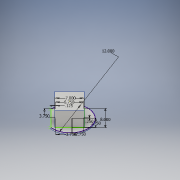
# Autodesk Inventor part: Hermes plate
Saved by Autodesk Inventor 2016 (Build 200138000, 138)
## iProperties
Created: 2016-12-06
Part Number: Hermes plate
Material: Aluminum 6061
Document SubType Name: Modeling
Designer: Ethan
Density: 2.7 g/cm^3
Appearance: Aluminum - Flat
Mass: 3970.64 g
Surface Area: 4553.61 cm^2
Volume: 1470.61 cm^3
Author: Ethan
Autodesk Inventor part; units mm, degrees
ref_plane "YZ Plane" through (0, 0, 0) normal (1, 0, 0) x (0, 1, 0)
ref_plane "XZ Plane" through (0, 0, 0) normal (0, 1, 0) x (-1, 0, 0)
ref_plane "XY Plane" through (0, 0, 0) normal (0, 0, 1) x (1, 0, 0)
sketch "Sketch1" plane through (0, 0, 0) normal (0, 1, 0) x (-1, 0, 0)
  arc A0 (13.4296, 151.8071) -> (151.8071, 13.4296) centre (0, 0) ccw
  line L0 (13.4296, 151.8071) -> (151.8071, 13.4296)
  dimension "d0" = 304.8
  constraints: 2 end point, 2 point on circle, 1 centre point, 1 coincident
  measures "d0" diameter of A0
sketch "Sketch2" plane through (0, 0, 0) normal (0, 1, 0) x (-1, 0, 0)
  line L0 (-4.2626, 135.0266) -> (-129.9862, 9.3031)
  line L1 (-129.9862, 9.3031) -> (13.6979, -134.381)
  line L2 (13.6979, -134.381) -> (139.4215, -8.6575)
  line L3 (139.4215, -8.6575) -> (-4.2626, 135.0266)
  line L4 (-4.2626, 135.0266) -> (-76.1046, 63.1846)
  line L5 (-76.1046, 63.1846) -> (-4.2626, -8.6575)
  line L6 (-4.2626, -8.6575) -> (67.5795, 63.1846)
  line L7 (67.5795, 63.1846) -> (-4.2626, 135.0266)
  line L8 (-129.9862, 9.3031) -> (-76.1046, 63.1846)
  line L9 (-76.1046, 63.1846) -> (-4.2626, -8.6575)
  line L10 (-4.2626, -8.6575) -> (-58.1441, -62.539)
  line L11 (-58.1441, -62.539) -> (-129.9862, 9.3031)
  line L12 (-4.2626, 130.5365) -> (-71.6145, 63.1846)
  line L13 (-71.6145, 63.1846) -> (-4.2626, -4.1673)
  line L14 (-4.2626, -4.1673) -> (63.0893, 63.1846)
  line L15 (63.0893, 63.1846) -> (-4.2626, 130.5365)
  line L16 (-125.496, 9.3031) -> (-76.1046, 58.6945)
  line L17 (-76.1046, 58.6945) -> (-8.7527, -8.6575)
  line L18 (-8.7527, -8.6575) -> (-58.1441, -58.0489)
  line L19 (-58.1441, -58.0489) -> (-125.496, 9.3031)
  line L20 (67.5795, 58.6945) -> (-53.654, -62.539)
  line L21 (-53.654, -62.539) -> (13.6979, -129.8909)
  line L22 (13.6979, -129.8909) -> (134.9314, -8.6575)
  line L23 (134.9314, -8.6575) -> (67.5795, 58.6945)
  point P0 (0, 0)
  point P1 (4.7177, 0.3228)
  dimension "d42" = 203.2
  dimension "d43" = 177.8
  dimension "d44" = 3.175
  dimension "d45" = 6.35
  dimension "d46" = 95.25
  dimension "d47" = 171.45
  dimension "d48" = 95.25
  dimension "d49" = 69.85
  dimension "d50" = 95.25
  constraints: 48 end point, 12 parallel, 6 perpendicular
  measures "d42" distance of L0.end L1.end
  measures "d43" distance of L1.end L2.end
  measures "d44" distance between parallel lines of L3 L23
  measures "d45" distance between parallel lines of L18 L20
  measures "d46" distance between parallel lines of L20 L22
  measures "d47" distance between parallel lines of L21 L23
  measures "d48" distance of L16.end L17.end
  measures "d49" distance of L17.end L18.end
  measures "d50" distance of L13.end L14.end
extrude "Extrusion1" add sketch "Sketch1" against normal blind 12.7
extrude "Extrusion2" add sketch "Sketch2" along normal blind 127
sketch "Sketch3" plane through (-13.6979, 0, -134.381) normal (0.7071068, 0, -0.7071068) x (-0.7071068, 0, -0.7071068)
  line L0 (-29.972, 4.7625) -> (-71.628, 4.7625)
  line L1 (-74.803, 7.9375) -> (-74.803, 49.5935)
  line L2 (-71.628, 52.7685) -> (-29.972, 52.7685)
  line L3 (-26.797, 49.5935) -> (-26.797, 7.9375)
  line L4 (-257.1076, 0) -> (47.6924, 0) projected
  line L5 (0, 0) -> (0, 127) projected
  arc A0 (-26.797, 49.5935) -> (-29.972, 52.7685) centre (-29.972, 49.5935) ccw
  arc A1 (-29.972, 4.7625) -> (-26.797, 7.9375) centre (-29.972, 7.9375) ccw
  arc A2 (-74.803, 7.9375) -> (-71.628, 4.7625) centre (-71.628, 7.9375) ccw
  arc A3 (-71.628, 52.7685) -> (-74.803, 49.5935) centre (-71.628, 49.5935) ccw
  point P0 (-104.7076, 0)
  point P1 (-74.803, 52.7685)
  point P2 (-74.803, 4.7625)
  point P3 (-26.797, 52.7685)
  point P4 (-6.8599, 0)
  point P5 (-202.5554, 0)
  dimension "d25" = 4.7625
  dimension "d26" = 48.006
  dimension "d27" = 26.797
  dimension "d28" = 48.006
  dimension "d29" = 3.175
  constraints: 8 end point, 8 point on circle, 8 tangent, 6 point on line, 4 centre point, 3 equal radius, 2 parallel, 1 horizontal, 1 perpendicular
  measures "d25" distance between parallel lines of L4 L0
  measures "d26" distance of point (-74.803, 52.768) point (-26.797, 52.769)
  measures "d27" distance between parallel lines of L5 L3
  measures "d28" distance of point (-74.803, 4.762) point (-74.803, 52.768)
  measures "d29" radius of A0
sketch "Sketch4" plane through (4.2626, 0, 135.0266) normal (-0.7071068, 0, 0.7071068) x (0.7071068, 0, 0.7071068)
  line L0 (-98.425, 52.7812) -> (-50.419, 52.7812)
  line L1 (-50.419, 52.7812) -> (-50.419, 4.7752)
  line L2 (-50.419, 4.7752) -> (-98.425, 4.7752)
  line L3 (-98.425, 4.7752) -> (-98.425, 52.7812)
  line L4 (-0.6446, 0) -> (-196.3401, 0) projected
  line L5 (0, 0) -> (0, 127) projected
  point P0 (-98.4924, 0)
  dimension "d30" = 48.006
  dimension "d31" = 48.006
  dimension "d32" = 4.7752
  dimension "d33" = 50.419
  constraints: 8 end point, 2 parallel, 1 horizontal, 1 perpendicular
  measures "d30" distance of L0.start L0.end
  measures "d31" distance of L2.end L0.start
  measures "d32" distance between parallel lines of L4 L2
  measures "d33" distance between parallel lines of L5 L1
extrude "Extrusion3" cut sketch "Sketch4" against normal up to next
extrude "Extrusion4" cut sketch "Sketch3" against normal up to next
sketch "Sketch5" plane through (0, 127, 0) normal (0, 1, 0) x (1, 0, 0)
  line L0 (-139.4215, 8.6575) -> (-13.6979, 134.381) projected
  line L1 (4.2626, -135.0266) -> (-139.4215, 8.6575)
  line L2 (-139.4215, 8.6575) -> (-13.6979, 134.381)
  line L3 (-13.6979, 134.381) -> (129.9862, -9.3031) projected
  line L4 (-13.6979, 134.381) -> (129.9862, -9.3031)
  line L5 (129.9862, -9.3031) -> (4.2626, -135.0266)
  point P0 (0, 0)
  constraints: 8 end point, 2 collinear, 2 perpendicular
extrude "Extrusion5" cut sketch "Sketch5" against normal blind 3.175
sketch "Sketch6" plane through (0, 123.825, 0) normal (0, 1, 0) x (1, 0, 0)
  line L0 (4.2626, -135.0266) -> (-139.4215, 8.6575) projected
  line L1 (4.2626, -135.0266) -> (-139.4215, 8.6575)
  line L2 (-139.4215, 8.6575) -> (-13.6979, 134.381)
  line L3 (-13.6979, 134.381) -> (129.9862, -9.3031) projected
  line L4 (-13.6979, 134.381) -> (129.9862, -9.3031)
  line L5 (129.9862, -9.3031) -> (4.2626, -135.0266)
  line L6 (4.2626, -130.5365) -> (71.6145, -63.1846) projected
  point P0 (0, 0)
  constraints: 8 end point, 2 collinear, 1 parallel, 1 perpendicular
extrude "Extrusion6" add sketch "Sketch6" along normal blind 3.175
sketch "Sketch7" plane through (0, 127, 0) normal (0, 1, 0) x (1, 0, 0)
  point P0 (0, 0)
body "Solid1"
